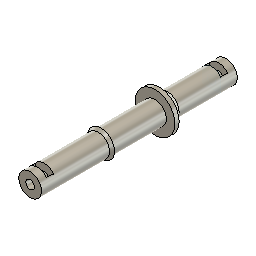
_Shaft.4d7b509e-9c09-4673-b3b6-3452699cbe1a (Autodesk Fusion 360 design; units mm, degrees)
Autodesk Fusion 360 part; units mm, degrees
sketch "Sketch1" plane through (0, 0, 0) normal (0, 0, 1) x (1, 0, 0)
  circle A0 centre (0, 0) radius 4
  circle A1 centre (0, 0) radius 1.5
  dimension "d1" = 8
  dimension "d2" = 3
  constraint coincident A0.centre A1.centre
  constraint concentric A0 A1
  measures "d1" diameter of A0
  measures "d2" diameter of A1
extrude "Extrude1" add sketch "Sketch1" along normal blind 12
sketch "Sketch2" plane through (0, 0, 12) normal (0, 0, 1) x (1, 0, 0)
  circle A0 centre (0, 0) radius 1.5
  circle A1 centre (0, 0) radius 4
extrude "Extrude2" add sketch "Sketch2" along normal blind 13 contours A0 | A1
ref_plane "WorkPlane1" through (0, 4, 3.3273) normal (0, 1, 0) x (1, 0, 0)
sketch "Sketch3" plane through (0, 4, 0) normal (0, 1, 0) x (1, 0, 0)
  line L0 (0, 0) -> (0, -2.6)
  line L1 (0, -5) -> (-3.1754, -5)
  line L2 (-3.1754, -5) -> (-3.1754, -2.6)
  line L3 (-3.1754, -2.6) -> (0, -2.6)
  line L4 (0, -5) -> (3.1754, -5)
  line L5 (3.1754, -5) -> (3.1754, -2.6)
  line L6 (3.1754, -2.6) -> (0, -2.6)
  dimension "d8" = 5
  dimension "d9" = 3.1754
  dimension "d10" = 2.4
  constraint coincident L0.start origin
  constraint vertical L0
  constraint perpendicular L0 L1
  constraint perpendicular L1 L2
  constraint perpendicular L0 L3
  constraint symmetric L1.start L0 L4.start
  constraint symmetric L0 L1.end L4.end
  constraint symmetric L0 L2.end L5.end
  measures "d8" distance of L0.start L1.start
  measures "d9" distance of L1.start L1.end
  measures "d10" distance of L1.end L2.end
extrude "Extrude3" cut sketch "Sketch3" against normal blind 6.75
sketch "Sketch4" plane through (0, 0, 12) normal (0, 0, -1) x (-1, 0, 0)
  arc A0 (-3.1754, -2.4325) -> (-2.9047, -2.75) centre (0, 0) ccw
  line L0 (-3.1754, 2.4325) -> (-3.1754, -2.4325)
  line L1 (-2.9047, -2.75) -> (2.9047, -2.75)
  line L2 (3.1754, -2.4325) -> (3.1754, 2.4325)
  line L3 (-3.1754, 0) -> (-1.5877, -2.75)
  line L4 (-1.5877, -2.75) -> (1.5877, -2.75)
  line L5 (1.5877, -2.75) -> (3.1754, 0)
  arc A1 (2.9047, -2.75) -> (3.1754, -2.4325) centre (0, 0) ccw
  arc A2 (-4, 0) -> (4, 0) centre (0, 0) ccw
  line L6 (-4, 0) -> (-3.1754, 0)
  line L7 (3.1754, 0) -> (4, 0)
  circle A3 centre (0, 0) radius 1.5
  arc A4 (3.1754, 2.4325) -> (-3.1754, 2.4325) centre (0, 0) ccw
  dimension "d13" = 3.1754
  constraint coincident A0.centre A1.centre
  constraint perpendicular L0 L6
  constraint collinear L6 L7
  measures "d13" distance of L5.end A0.centre
extrude "Extrude4" add sketch "Sketch4" along normal blind 2.4 contours A0 L0 L1 L3 A2 | L0 A2 L6 | L1 L4 A2 | L1 L2 L5 A1 A2
sketch "Sketch5" plane through (0, 0, 25) normal (0, 0, 1) x (1, 0, 0)
  circle A0 centre (0, 0) radius 4
  circle A1 centre (0, 0) radius 7
  dimension "d16" = 14
  constraint coincident A0.centre A1.centre
  measures "d16" diameter of A1
extrude "Extrude5" add sketch "Sketch5" against normal blind 1.5
sketch "Sketch6" plane through (0, 0, 25) normal (0, 0, 1) x (1, 0, 0)
  circle A0 centre (0, 0) radius 7
  circle A1 centre (0, 0) radius 4
  dimension "d19" = 8
  constraint coincident A0.centre A1.centre
  measures "d19" diameter of A1
extrude "Extrude6" add sketch "Sketch6" along normal blind 19.05 contours A1
ref_plane "WorkPlane2" through (0, 0, 34.525) normal (0, 0, 1) x (1, 0, 0)
chamfer "Chamfer1" distance 3 angle 45 1 edges at (-3.7293, 1.4465, 23.5)
ref_plane "WorkPlane3" through (0, 0, 44.05) normal (0, 0, 1) x (1, 0, 0)
mirror "Mirror1" about plane through (0, 0, 34.525) normal (0, 0, 1) of bodies 1 merged
sketch "Sketch7" plane through (0, 0, 44.05) normal (0, 0, 1) x (1, 0, 0)
  circle A0 centre (0, 0) radius 10.4439
  circle A1 centre (0, 0) radius 4
  dimension "d26" = 8
  constraint coincident A0.centre A1.centre
  measures "d26" diameter of A1
extrude "Extrude7" cut sketch "Sketch7" along normal blind 26
sketch "Sketch8" plane through (0, 0, 34.525) normal (0, 0, 1) x (1, 0, 0)
sketch "Sketch9" plane through (0, 0, 44.05) normal (0, 0, 1) x (1, 0, 0)
  circle A0 centre (0, 0) radius 4.75
  circle A1 centre (0, 0) radius 4
  dimension "d29" = 9.5
  dimension "d30" = 8
  constraint coincident A0.centre A1.centre
  measures "d29" diameter of A0
  measures "d30" diameter of A1
extrude "Extrude8" add sketch "Sketch9" along normal blind 1
chamfer "Chamfer2" distance 0.75 distance2 1 1 edges at (-4.4286, -1.7177, 45.05) measured on face at (4.4674, -0.4347, 45.05)
sketch "Sketch10" plane through (0, 0, 5) normal (0, 0, -1) x (-1, 0, 0)
  circle A0 centre (0, 0) radius 1.5
  arc A1 (-3.1754, -2.4325) -> (-2.9047, -2.75) centre (0, 0) ccw
  line L0 (-2.9047, -2.75) -> (2.9047, -2.75)
  arc A2 (2.9047, -2.75) -> (3.1754, -2.4325) centre (0, 0) ccw
  line L1 (3.1754, -2.4325) -> (3.1754, 2.4325)
  arc A3 (3.1754, 2.4325) -> (-3.1754, 2.4325) centre (0, 0) ccw
  line L2 (-3.1754, 2.4325) -> (-3.1754, -2.4325)
sketch "Sketch11" plane through (0, 0, 12) normal (0, 0, -1) x (1, 0, 0)
sketch "Sketch12" plane through (0, 0, 5) normal (0, 0, -1) x (-1, 0, 0)
  line L0 (-2.9047, -2.75) -> (2.9047, -2.75)
  arc A0 (3.1754, 2.4325) -> (-3.1754, 2.4325) centre (0, 0) ccw
  line L1 (-3.1754, 2.4325) -> (-3.1754, -2.4325)
  line L2 (3.1754, 0) -> (4, 0)
  arc A1 (-4, 0) -> (4, 0) centre (0, 0) ccw
  line L3 (-3.1754, 0) -> (-1.5877, -2.75)
  circle A2 centre (0, 0) radius 1.5
  arc A3 (2.9047, -2.75) -> (3.1754, -2.4325) centre (0, 0) ccw
  line L4 (-4, 0) -> (-3.1754, 0)
  line L5 (-1.5877, -2.75) -> (1.5877, -2.75)
  line L6 (3.1754, -2.4325) -> (3.1754, 2.4325)
  arc A4 (-3.1754, -2.4325) -> (-2.9047, -2.75) centre (0, 0) ccw
  line L7 (1.5877, -2.75) -> (3.1754, 0)
  dimension "d35" = 3.1754
  constraint coincident A0.centre A1.centre
  constraint perpendicular L1 L4
  constraint collinear L2 L4
  measures "d35" distance of L2.start A0.centre
extrude "Extrude9" add sketch "Sketch12" along normal blind 4.5 contours L0 L1 A1 L3 A4 | L0 A1 L5 | L0 A1 A3 L6 L7 | L2 A1 L6
mirror "Mirror2" about plane through (0, 0, 34.525) normal (0, 0, 1) of "Extrude9"
